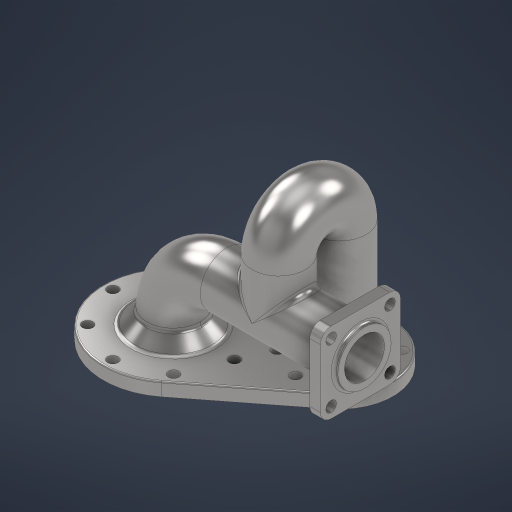
# Autodesk Inventor part: 3D MODEL
Saved by Autodesk Inventor 2023 (Build 270158000, 158)
## iProperties
Created: 2023-12-27
Part Number: 3D MODEL
Material: Steel, Alloy
Document SubType Name: Modeling
Designer: User
Density: 7.73 g/cm^3
Appearance: Semi-Polished
Author: User
Autodesk Inventor part; units mm, degrees
ref_plane "YZ Plane" through (0, 0, 0) normal (1, 0, 0) x (0, 1, 0)
ref_plane "XY Plane" through (0, 0, 0) normal (0, 0, 1) x (1, 0, 0)
sketch "Sketch1" plane through (0, 0, 0) normal (0, 0, 1) x (1, 0, 0)
  arc A0 (-27.097, -44.9667) -> (-32.2465, 41.4296) centre (0, 0) ccw
  arc A1 (-103.3771, -13.9346) -> (-39.1564, -50.7656) centre (-78.8083, -45.5) ccw
  line L0 (0, 0) -> (-78.8083, -45.5) construction
  line L1 (-171.1943, 0) -> (93.3182, 0) construction
  line L2 (-103.3771, -13.9346) -> (-32.2465, 41.4296)
  arc A2 (-27.097, -44.9667) -> (-39.1564, -50.7656) centre (-31.226, -51.8188) ccw
  circle A3 centre (-78.8083, -45.5) radius 33 construction
  circle A4 centre (0, 0) radius 45.5 construction
  circle A5 centre (0, 45.5) radius 4
  circle A6 centre (-78.8083, -12.5) radius 4
  circle A7 centre (-102.1428, -22.1655) radius 4
  circle A8 centre (-111.8083, -45.5) radius 4
  circle A9 centre (-102.1428, -68.8345) radius 4
  circle A10 centre (-78.8083, -78.5) radius 4
  circle A11 centre (-55.4738, -68.8345) radius 4
  circle A12 centre (-45.8083, -45.5) radius 4
  circle A13 centre (-55.4738, -22.1655) radius 4
  circle A14 centre (-32.1734, 32.1734) radius 4
  circle A15 centre (-45.5, 0) radius 4
  circle A16 centre (-32.1734, -32.1734) radius 4
  circle A17 centre (0, -45.5) radius 4
  circle A18 centre (32.1734, -32.1734) radius 4
  circle A19 centre (45.5, 0) radius 4
  circle A20 centre (32.1734, 32.1734) radius 4
  circle A21 centre (-78.8083, -45.5) radius 15
  circle A22 centre (0, 0) radius 37
  circle A23 centre (0, 0) radius 15
  dimension "d11" = 91
  dimension "d12" = 66
  dimension "d2" = 30
  dimension "d4" = 91
  dimension "d5" = 52.5
  dimension "d6" = 40
  dimension "d8" = 8
  dimension "d13" = 8
  dimension "d14" = 8
  dimension "d17" = 360
  dimension "d21" = 360
  dimension "d26" = 74
  dimension "d27" = 30
  dimension "d28" = 30
  constraints: 22 centre point, 6 coincident, 6 point on circle, 4 end point, 4 tangent, 4 vertical alignment, 38 other
  measures "d2" angle of L1 L0
  measures "d4" distance of L0.start L0.end
  measures "d5" radius of A0
  measures "d6" radius of A1
  measures "d8" radius of A2
  measures "d13" diameter of A5
  measures "d14" diameter of A6
  measures "d26" diameter of A22
  measures "d27" diameter of A23
  measures "d28" diameter of A21
extrude "Extrusion1" add sketch "Sketch1" along normal blind 10 contours A2 A1 L2 A0 | A22
extrude "Extrusion2" cut sketch "Sketch1" along normal blind 4 contours A22
sketch "Sketch2" plane through (0, 0, 0) normal (0, 1, 0) x (-1, 0, 0)
  line L0 (-20, 20) -> (20, 20)
  line L1 (37, 0) -> (-37, 0) projected
  line L2 (-20, 20) -> (-36, 4)
  line L3 (37, 4) -> (-37, 4) projected
  line L4 (20, 20) -> (36, 4)
  line L5 (0, 20) -> (0, 4)
  line L6 (-15, 4) -> (15, 4) projected
  line L7 (-15, 20) -> (-31, 4)
  line L8 (15, 20) -> (31, 4)
  point P0 (0, 0)
  point P1 (0, 0)
  point P2 (0, 4)
  dimension "d33" = 40
  dimension "d34" = 20
  dimension "d35" = 90
  dimension "d36" = 15
  constraints: 12 end point, 6 point on line, 3 midpoint, 1 horizontal, 1 parallel, 1 vertical alignment, 2 other
  measures "d33" distance of L0.start L0.end
  measures "d34" distance between parallel lines of L0 L1
  measures "d35" angle of L4 L2
  measures "d36" distance from line of L5 L7.start
revolve "Revolution1" cut sketch "Sketch2" angle 360 about axis through (0, 0, 20) along (0, 0, -1) contours L0 L8 L3 L5
revolve "Revolution2" add sketch "Sketch2" angle 360 about axis through (0, 0, 20) along (0, 0, -1) contours L0 L4 L3 L8
sketch "Sketch3" plane through (0, 0, 0) normal (0, 1, 0) x (-1, 0, 0)
  line L0 (15, 20) -> (-15, 20) construction
  arc A0 (40, 60) -> (0, 20) centre (40, 20) ccw
  line L1 (40, 60) -> (143, 60)
  line L2 (32.2465, 0) -> (-52.5, 0) construction
  point P0 (0, 0)
  point P1 (27.097, 0)
  dimension "d39" = 60
  dimension "d40" = 143
  dimension "d41" = 40
  constraints: 2 end point, 2 point on circle, 1 centre point, 1 horizontal, 1 line through centre, 1 midpoint, 1 tangent
  measures "d39" distance between parallel lines of L1 L2
  measures "d40" horizontal distance of L1.end point (0, 0)
  measures "d41" radius of A0
sketch "Sketch4" plane through (0, 0, 20) normal (0, 0, 1) x (1, 0, 0)
  circle A0 centre (0, 0) radius 15 projected
  circle A1 centre (0, 0) radius 20 projected
sweep "Sweep1" add profiles "Sketch4" path "Sketch3"
ref_plane "Work Plane1" through (-140, 0, 60) normal (-1, 0, 0) x (0, 0, 1)
sketch "Sketch5" plane through (-140, 0, 60) normal (-1, 0, 0) x (0, 0, 1)
  circle A0 centre (0, 0) radius 15 construction
  circle A1 centre (0, 0) radius 20 projected
  line L0 (22, 30) -> (-22, 30)
  line L1 (-30, 22) -> (-30, -22)
  line L2 (-22, -30) -> (22, -30)
  line L3 (30, -22) -> (30, 22)
  line L4 (30, 30) -> (-30, -30) construction
  line L5 (-30, 30) -> (30, -30) construction
  arc A2 (-22, 30) -> (-30, 22) centre (-22, 22) ccw
  arc A3 (-30, -22) -> (-22, -30) centre (-22, -22) ccw
  arc A4 (22, -30) -> (30, -22) centre (22, -22) ccw
  arc A5 (30, 22) -> (22, 30) centre (22, 22) ccw
  circle A6 centre (22, 22) radius 4
  circle A7 centre (22, -22) radius 4
  circle A8 centre (-22, -22) radius 4
  circle A9 centre (-22, 22) radius 4
  point P0 (-60, 0)
  dimension "d45" = 60
  dimension "d46" = 60
  dimension "d47" = 8
  dimension "d48" = 8
  constraints: 12 end point, 8 centre point, 8 point on circle, 8 point on line, 8 tangent, 6 equal radius, 4 coincident, 2 midpoint, 2 parallel, 1 horizontal, 1 perpendicular
  measures "d45" distance of L5.end L4.end
  measures "d46" distance of L4.end L5.start
  measures "d47" radius of A2
  measures "d48" diameter of A6
extrude "Extrusion3" add sketch "Sketch5" against normal blind 8
ref_plane "Work Plane2" through (-78.8083, -45.5, 0) normal (-1, 0, 0) x (0, 0, 1)
sketch "Sketch6" plane through (-78.8083, -45.5, 0) normal (-1, 0, 0) x (0, 0, 1)
  circle A0 centre (60, 45.5) radius 20 construction
  line L0 (10, 15) -> (10, -15) construction
  line L1 (60, 45.5) -> (95, 45.5)
  arc A1 (95, 0) -> (95, 45.5) centre (95, 22.75) ccw
  line L2 (95, 0) -> (10, 0)
  line L3 (0, 15) -> (0, -15) projected
  point P0 (0, 45.5)
  dimension "d52" = 60
  dimension "d55" = 22.75
  dimension "d56" = 95
  constraints: 4 end point, 2 point on circle, 2 tangent, 1 centre point, 1 horizontal, 1 midpoint
  measures "d52" distance of L1.start point (0, 45.5)
  measures "d55" radius of A1
  measures "d56" distance from line of A1.centre L3
sketch "Sketch7" plane through (0, 0, 10) normal (0, 0, 1) x (1, 0, 0)
  circle A0 centre (-78.8083, -45.5) radius 15 projected
  circle A1 centre (-78.8083, -45.5) radius 20
  point P0 (0, 0)
  dimension "d57" = 40
  constraints: 1 centre point, 1 coincident
  measures "d57" diameter of A1
sweep "Sweep2" add profiles "Sketch7" path "Sketch6" path curves L2 A1 L1
delete faces "Delete Face1" heal yes whole lump no faces at (-98.8083, 0, 65) (-97.0075, -0.6027, 60) (-93.8083, 0, 65) (-63.8083, 0, 65)
delete faces "Delete Face2" heal yes whole lump no faces at (-83.3954, 4.9799, 79.3701)
fillet "Fillet1" radius 4 9 edges at (30, 0, 10) (0, 20, 20) (0, -20, 20) (-98.8083, -45.5, 10) (-92.9504, 14.1421, 74.1421) (-92.9504, -14.1421, 74.1421) (-64.6662, 14.1421, 74.1421) (-64.6662, -14.1421, 74.1421) (-132, 0, 40)
fillet "Fillet2" radius 1 4 edges at (-34.6929, -44.609, 10) (52.407, 3.1237, 10) (-67.8118, 13.7475, 10) (-98.7082, -80.1986, 10)
fillet "Fillet3" radius 2 1 edges at (-140, 0, 40)
body "Solid1"
